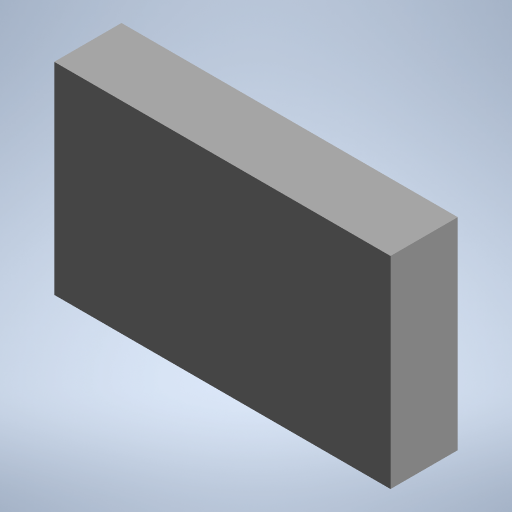
# Autodesk Inventor part: 이니셜
Saved by Autodesk Inventor 2024 (Build 280153020, 153B)
## iProperties
Part Number: 이니셜
Material: 일반
Document SubType Name: 모델링
Designer: admin
Appearance: 기본값
Author: admin
Autodesk Inventor part; units mm, degrees
ref_plane "YZ 평면" through (0, 0, 0) normal (1, 0, 0) x (0, 1, 0)
ref_plane "XZ 평면" through (0, 0, 0) normal (0, 1, 0) x (-1, 0, 0)
ref_plane "XY 평면" through (0, 0, 0) normal (0, 0, 1) x (1, 0, 0)
sketch "스케치1" plane through (0, 0, 0) normal (0, 0, 1) x (1, 0, 0)
  line L0 (0, 0) -> (50, 0)
  line L1 (50, 0) -> (50, 30)
  line L2 (50, 30) -> (0, 30)
  line L3 (0, 30) -> (0, 0)
  constraints: 8 end point, 2 parallel, 1 horizontal, 1 perpendicular
extrude "돌출1" add sketch "스케치1" along normal blind 10
sketch "스케치2" plane through (0, 0, 0) normal (0, 0, -1) x (-1, 0, 0)
  spline S0 degree 2 poles (-33.9271, 18.5737) (-33.9271, 17.4068) (-34.7585, 15.3063) (-35.5024, 14.577) knots 0 0 0 1 2 2 2
  spline S1 degree 2 poles (-35.5024, 14.577) (-36.436, 13.658) (-38.9595, 12.7099) (-40.8849, 12.7099) knots 0 0 0 1 2 2 2
  line L0 (-40.8849, 12.7099) -> (-42.9125, 12.7099)
  line L1 (-42.9125, 12.7099) -> (-42.9125, 6)
  line L2 (-42.9125, 6) -> (-45.3047, 6)
  line L3 (-45.3047, 6) -> (-45.3047, 24)
  line L4 (-45.3047, 24) -> (-40.7828, 24)
  spline S2 degree 2 poles (-40.7828, 24) (-39.1783, 24) (-36.9319, 23.4749) (-36.0713, 22.8768) knots 0 0 0 1 2 2 2
  spline S3 degree 2 poles (-36.0713, 22.8768) (-35.0648, 22.1912) (-33.9271, 20.0762) (-33.9271, 18.5737) knots 0 0 0 1 2 2 2
  spline S4 degree 2 poles (-36.4214, 18.5008) (-36.4214, 19.4344) (-37.0632, 20.8055) (-37.7196, 21.2431) knots 0 0 0 1 2 2 2
  spline S5 degree 2 poles (-37.7196, 21.2431) (-38.2885, 21.6224) (-39.8055, 21.9287) (-40.9287, 21.9287) knots 0 0 0 1 2 2 2
  line L5 (-40.9287, 21.9287) -> (-42.9125, 21.9287)
  line L6 (-42.9125, 21.9287) -> (-42.9125, 14.752)
  line L7 (-42.9125, 14.752) -> (-41.2788, 14.752)
  spline S6 degree 2 poles (-41.2788, 14.752) (-39.8201, 14.752) (-38.0259, 15.2188) (-37.4425, 15.8314) knots 0 0 0 1 2 2 2
  spline S7 degree 2 poles (-37.4425, 15.8314) (-36.9028, 16.3712) (-36.4214, 17.6402) (-36.4214, 18.5008) knots 0 0 0 1 2 2 2
  line L8 (-31.6515, 6) -> (-31.6515, 24)
  line L9 (-31.6515, 24) -> (-20.3906, 24)
  line L10 (-20.3906, 24) -> (-20.3906, 21.8703)
  line L11 (-20.3906, 21.8703) -> (-29.2593, 21.8703)
  line L12 (-29.2593, 21.8703) -> (-29.2593, 16.94)
  line L13 (-29.2593, 16.94) -> (-20.9887, 16.94)
  line L14 (-20.9887, 16.94) -> (-20.9887, 14.8104)
  line L15 (-20.9887, 14.8104) -> (-29.2593, 14.8104)
  line L16 (-29.2593, 14.8104) -> (-29.2593, 8.1297)
  line L17 (-29.2593, 8.1297) -> (-20.3906, 8.1297)
  line L18 (-20.3906, 8.1297) -> (-20.3906, 6)
  line L19 (-20.3906, 6) -> (-31.6515, 6)
  line L20 (-4.6953, 6) -> (-7.0875, 6)
  line L21 (-7.0875, 6) -> (-7.0875, 14.8104)
  line L22 (-7.0875, 14.8104) -> (-15.3728, 14.8104)
  line L23 (-15.3728, 14.8104) -> (-15.3728, 6)
  line L24 (-15.3728, 6) -> (-17.765, 6)
  line L25 (-17.765, 6) -> (-17.765, 24)
  line L26 (-17.765, 24) -> (-15.3728, 24)
  line L27 (-15.3728, 24) -> (-15.3728, 16.94)
  line L28 (-15.3728, 16.94) -> (-7.0875, 16.94)
  line L29 (-7.0875, 16.94) -> (-7.0875, 24)
  line L30 (-7.0875, 24) -> (-4.6953, 24)
  line L31 (-4.6953, 24) -> (-4.6953, 6)
  point P0 (0, 0)
  point P1 (0, 0)
  point P2 (-25, 15)
  dimension "d2" = 25
  dimension "d3" = 15
  constraints: 1 coincident, 1 other
  measures "d2" horizontal distance of point (0, 0) point (-25, 15)
  measures "d3" vertical distance of point (0, 0) point (-25, 15)
emboss "엠보싱1" sketch "스케치2" operation cut depth 5 direction (0, 0, 1)
